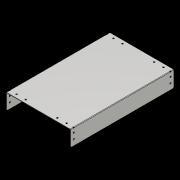
# Autodesk Inventor part: top
Saved by Autodesk Inventor 2018.2 (Build 222227000, 227)
## iProperties
Created: 2019-11-17
Part Number: top
Material: アルミニウム 6061
Document SubType Name: Sheet Metal
Designer: gisen
Density: 2.7 g/cm^3
Sheet Metal Rule: Default_mm
Appearance: アルミニウム - フラット
Author: gisen
Autodesk Inventor part; units mm, degrees
ref_plane "YZ Plane" through (0, 0, 0) normal (1, 0, 0) x (0, 1, 0)
ref_plane "XZ Plane" through (0, 0, 0) normal (0, 1, 0) x (-1, 0, 0)
ref_plane "XY Plane" through (0, 0, 0) normal (0, 0, 1) x (1, 0, 0)
sketch "スケッチ1" plane through (0, 0, 0) normal (0, 0, 1) x (1, 0, 0)
  line L0 (-67.5, -110) -> (67.5, -110)
  line L1 (67.5, -110) -> (67.5, 110)
  line L2 (67.5, 110) -> (-67.5, 110)
  line L3 (-67.5, 110) -> (-67.5, -110)
  line L4 (-67.5, -110) -> (67.5, 110) construction
  line L5 (67.5, -110) -> (-67.5, 110) construction
  point P0 (0, 0)
  dimension "d0" = 135
  dimension "d1" = 220
  measures "d0" distance of L2.end L1.end
  measures "d1" distance of L1.end L0.end
extrude "プレート1" add sketch "スケッチ1" along normal blind 1
sketch "スケッチ2" plane through (67.501, -110, -0.001) normal (1, 0, 0) x (0, 1, 0)
  line L0 (220, 0) -> (0, 0)
  line L1 (0, 0) -> (0, -32.999)
  line L2 (0, -32.999) -> (220, -32.999)
  line L3 (220, -32.999) -> (220, 0)
  constraints: 6 end point, 1 horizontal, 1 perpendicular, 1 vertical
edge flange "フランジ1" height 33 angle 90 thickness 1 bend radius 0 thickness toward (1, 0, 0) relief straight relief width 1 relief depth 0.5 corner gap 0 corner form 0 edges at (67.5, 0, 0) (-67.5, 0, 0) wall of the first edge with corners at (67.501, 110, -0.001) (67.501, -110, -0.001) (67.501, -110, -33) (67.501, 110, -33)
bend "曲げ1"
corner "コーナー1"
sketch "スケッチ3" plane through (0, 0, 1) normal (0, 0, 1) x (1, 0, 0)
  line L0 (-67.5, -110) -> (-67.5, 110) construction
  line L1 (67.5, -110) -> (-67.5, -110) construction
  line L2 (67.5, 110) -> (67.5, -110) construction
  line L3 (-67.5, 110) -> (67.5, 110) construction
  line L4 (-67.5, 110) -> (-67.5, -110) construction
  line L5 (-67.5, 0) -> (67.5, 0) construction
  line L6 (67.5, -110) -> (67.5, 110) construction
  line L7 (67.5, -103) -> (-67.5, -103) construction
  line L8 (0, -110) -> (0, 110) construction
  line L9 (67.5, 110) -> (-67.5, 110) construction
  circle A0 centre (-33.75, -103) radius 1.6
  circle A1 centre (-53.25, -103) radius 1.6
  circle A2 centre (33.75, -103) radius 1.6
  circle A3 centre (53.25, -103) radius 1.6
  circle A4 centre (-33.75, 103) radius 1.6
  circle A5 centre (-53.25, 103) radius 1.6
  circle A6 centre (53.25, 103) radius 1.6
  circle A7 centre (33.75, 103) radius 1.6
  point P0 (0, 0)
  dimension "d13" = 7
  dimension "d14" = 3.2
  dimension "d15" = 19.5
  dimension "d16" = 33.75
  constraints: 8 centre point, 6 end point, 6 symmetric about line, 4 midpoint, 4 point on line, 1 equal radius, 1 perpendicular, 6 other
  measures "d13" distance between parallel lines of L1 L7
  measures "d14" diameter of A0
  measures "d15" distance of A0.centre A1.centre
  measures "d16" distance from line of L8 A0.centre
extrude "押し出し1" cut sketch "スケッチ3" against normal through all
sketch "スケッチ4" plane through (68.501, -110, -33) normal (1, 0, 0) x (0, 0, -1)
  line L0 (0, 220) -> (0, 0) construction
  line L1 (-33, 214.6) -> (-33, 211.4) construction
  line L2 (-33, 214.6) -> (-33, 211.4) construction
  line L3 (-33, 8.6) -> (-33, 5.4) construction
  line L4 (-33, 8.6) -> (-33, 5.4) construction
  line L5 (-33, 8.6) -> (-33, 5.4) construction
  line L6 (-33, 8.6) -> (-33, 5.4) construction
  line L7 (-33, 214.6) -> (-33, 211.4) construction
  line L8 (-33, 214.6) -> (-33, 211.4) construction
  line L9 (-33, 220) -> (-33, 0) construction
  line L10 (-33, 0) -> (-33, 220) construction
  line L11 (-33, 110) -> (0, 110) construction
  line L12 (0, 213) -> (-33, 213) construction
  line L13 (-33, 0) -> (-33, 220) construction
  line L14 (-32.999, 220) -> (0, 220) construction
  circle A0 centre (-24, 213) radius 1.6
  circle A1 centre (-12, 213) radius 1.6
  circle A2 centre (-24, 7) radius 1.6
  circle A3 centre (-12, 7) radius 1.6
  dimension "d19" = 7
  dimension "d20" = 3.2
  dimension "d21" = 12
  dimension "d22" = 9
  constraints: 4 centre point, 4 end point, 3 point on line, 2 symmetric about line, 1 equal radius, 1 midpoint, 1 perpendicular, 4 other
  measures "d19" distance between parallel lines of L12 L14
  measures "d20" diameter of A0
  measures "d21" distance of A1.centre A0.centre
  measures "d22" distance from line of A0.centre L10
extrude "押し出し2" cut sketch "スケッチ4" against normal through all
fillet "フィレット1" radius 3 4 edges at (68.001, 110, -33) (-68.001, 110, -33) (68.001, -110, -33) (-68.001, -110, -33)
unfold all bends "展開1" k factor 0.44 fixed face at (11.0609, -33.8347, 1)
sketch "スケッチ5" plane through (0, 0, 1) normal (0, 0, 1) x (1, 0, 0)
  line L0 (-68.1927, -110) -> (-68.1927, 110) construction
  line L1 (-67.5, -110) -> (-68.1927, -110) construction
  line L2 (-67.5, -110) -> (-67.5, 110) construction
  line L3 (-68.1927, 110) -> (-67.5, 110) construction
  line L4 (68.1927, 110) -> (68.1927, -110) construction
  line L5 (67.5, 110) -> (68.1927, 110) construction
  line L6 (67.5, 110) -> (67.5, -110) construction
  line L7 (68.1927, -110) -> (67.5, -110) construction
  line L8 (-67.5, 0) -> (67.5, 0) construction
  line L9 (-67.5, 110) -> (67.5, 110) construction
  line L10 (0, 110) -> (0, -110) construction
  line L11 (-68.1927, 110) -> (-67.5, 110) construction
  line L12 (-67.8464, 110) -> (-67.8464, -110) construction
  line L13 (-68.1927, -110) -> (-67.5, -110) construction
  circle A0 centre (-77.1917, 103) radius 1.6 construction
  circle A1 centre (-53.25, 103) radius 1.6 construction
  line L14 (-77.1917, 103) -> (-53.25, 103) construction
  circle A2 centre (-67.8464, 103) radius 1.1
  circle A3 centre (67.8464, 103) radius 1.1
  circle A4 centre (-67.8464, -103) radius 1.1
  circle A5 centre (67.8464, -103) radius 1.1
  point P0 (0, 0)
  dimension "d26" = 2.2
  constraints: 8 end point, 5 midpoint, 4 centre point, 3 symmetric about line, 2 point on line, 1 horizontal, 1 vertical, 3 other
  measures "d26" diameter of A2
extrude "押し出し3" cut sketch "スケッチ5" against normal up to surface (1 mm away)
refold all bends "再折り曲げ1"
equation "\"d2\" = Thickness"
equation "\"d3\" = BendReliefWidth"
equation "\"d4\" = BendReliefDepth"
equation "\"d5\" = MinimumRemnant"
equation "\"d10\" = CornerReliefSize"
equation "\"d11\" = GapSize"
equation "\"BendReliefWidth\" = Thickness"
equation "\"BendReliefDepth\" = 0.5 * Thickness"
equation "\"CornerReliefSize\" = 4 * Thickness"
equation "\"MinimumRemnant\" = 2 * Thickness"
equation "\"GapSize\" = Thickness"
equation "\"Thickness\" = 1"
